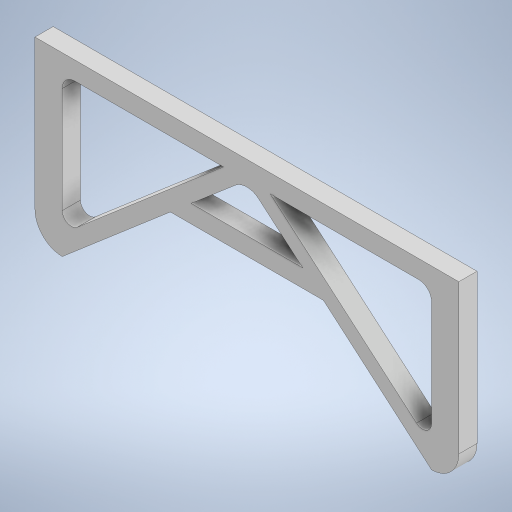
# Autodesk Inventor part: упрочнение
Saved by Autodesk Inventor 2023.1 (Build 271208000, 208)
## iProperties
Created: 2023-03-01
Part Number: упрочнение
Material: Типовые
Document SubType Name: Modeling
Designer: User
Density: 1 g/cm^3
Appearance: По умолчанию
Author: User
Autodesk Inventor part; units mm, degrees
ref_plane "YZ Plane" through (0, 0, 0) normal (1, 0, 0) x (0, 1, 0)
ref_plane "XZ Plane" through (0, 0, 0) normal (0, 1, 0) x (-1, 0, 0)
ref_plane "XY Plane" through (0, 0, 0) normal (0, 0, 1) x (1, 0, 0)
sketch "Эскиз1" plane through (0, 0, 0) normal (0, 0, 1) x (1, 0, 0)
  line L0 (-101.5, 0) -> (-101.5, 0)
  line L1 (-101.5, 21.8766) -> (-101.5, 80)
  line L2 (101.5, 80) -> (101.5, 21.8766)
  line L3 (101.5, 0) -> (101.5, 0)
  line L4 (116.5, 15) -> (116.5, 97)
  line L5 (116.5, 97) -> (-116.5, 97)
  line L6 (-116.5, 97) -> (-116.5, 15)
  line L7 (0, -23.1279) -> (0, 117.0213) projected
  arc A0 (-94.5, 87) -> (-101.5, 80) centre (-94.5, 80) ccw
  arc A1 (101.5, 80) -> (94.5, 87) centre (94.5, 80) ccw
  line L8 (-93.246, 18.0803) -> (-12.8397, 87)
  line L9 (12.8397, 87) -> (93.246, 18.0803)
  line L10 (-94.5, 87) -> (-12.8397, 87)
  line L11 (12.8397, 87) -> (94.5, 87)
  line L12 (-116.5, 0) -> (-101.5, 0)
  line L13 (101.5, 0) -> (116.5, 0)
  arc A2 (-116.5, 15) -> (-101.5, 0) centre (-101.5, 15) ccw
  arc A3 (101.5, 0) -> (116.5, 15) centre (101.5, 15) ccw
  arc A4 (-101.5, 21.8766) -> (-93.246, 18.0803) centre (-96.5, 21.8766) ccw
  arc A5 (93.246, 18.0803) -> (101.5, 21.8766) centre (96.5, 21.8766) ccw
  line L14 (-30.6646, 60.716) -> (30.6646, 60.716)
  line L15 (42.072, 50.9383) -> (-42.072, 50.9383)
  line L16 (-101.5, 0) -> (-42.072, 50.9383)
  line L17 (-30.6646, 60.716) -> (0, 87)
  line L18 (0, 87) -> (30.6646, 60.716)
  line L19 (42.072, 50.9383) -> (101.5, 0)
  point P0 (0, 0)
  dimension "d0" = 15
  dimension "d1" = 97
  dimension "d3" = 15
  dimension "d4" = 233
  dimension "d5" = 7
  dimension "d8" = 15
  dimension "d9" = 5
  constraints: 38 end point, 14 tangent, 12 point on circle, 9 perpendicular, 6 centre point, 5 point on line, 3 equal radius, 2 collinear, 2 horizontal, 2 horizontal alignment, 1 parallel, 1 other
  measures "d0" distance between parallel lines of L6 L1
  measures "d1" distance between parallel lines of L5 L0
  measures "d3" distance between parallel lines of L4 L2
  measures "d4" distance between parallel lines of L4 L6
  measures "d5" radius of A0
  measures "d8" radius of A2
  measures "d9" radius of A4
extrude "Выдавливание1" add sketch "Эскиз1" along normal blind 10 contours A3 L19 L15 L7 L14 L18 L5 L4 | L7 L17 L14 L15 L16 A2 L6 L5
fillet "Сопряжение1" radius 10 1 edges at (0, 87, 5)
